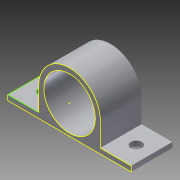
# Autodesk Inventor part: bearing mount
Saved by Autodesk Inventor 2013 (Build 170138000, 138)
## iProperties
Created: 2013-02-03
Part Number: bearing mount
Material: Aluminum 6061
Document SubType Name: Modeling
Designer: Arpan
Density: 2.71 g/cm^3
Mass: 38.247 g
Surface Area: 89.6456 cm^2
Volume: 14.1133 cm^3
Author: Arpan
Autodesk Inventor part; units mm, degrees
ref_plane "YZ Plane" through (0, 0, 0) normal (1, 0, 0) x (0, 1, 0)
ref_plane "XZ Plane" through (0, 0, 0) normal (0, 1, 0) x (-1, 0, 0)
ref_plane "XY Plane" through (0, 0, 0) normal (0, 0, 1) x (1, 0, 0)
sketch "Sketch1" plane through (0, 0, 0) normal (0, 0, 1) x (1, 0, 0)
  line L0 (0, 0) -> (-38.1, 0)
  line L1 (0, 0) -> (38.1, 0)
  line L2 (38.1, 0) -> (38.1, 3.175)
  line L3 (38.1, 3.175) -> (-38.1, 3.175)
  line L4 (-38.1, 3.175) -> (-38.1, 0)
  line L5 (0, 0) -> (0, 17.4625)
  circle A0 centre (0, 17.4625) radius 15.875
  arc A1 (7.6134, 0) -> (-7.6134, 0) centre (0, 17.4625) ccw
  line L6 (-19.05, 17.4625) -> (-19.05, 3.175)
  line L7 (19.05, 17.4625) -> (19.05, 3.175)
  dimension "d0" = 38.1
  dimension "d1" = 38.1
  dimension "d2" = 3.175
  dimension "d3" = 17.4625
  dimension "d4" = 31.75
  dimension "d5" = 3.175
  constraints: 16 end point, 4 perpendicular, 4 point on circle, 4 point on line, 2 centre point, 2 parallel, 2 tangent, 1 coincident, 1 collinear, 1 horizontal
  measures "d0" distance of L0.start L0.end
  measures "d1" distance of L0.start L1.end
  measures "d2" distance of L1.end L2.end
  measures "d3" distance of L0.start L5.end
  measures "d4" diameter of A0
  measures "d5" radial gap between concentric circles of A0 A1
extrude "Extrusion1" add sketch "Sketch1" along normal blind 25.4 contours L5 A0 L3 A1 L1 | L0 A1 L3 A0 L5 | L0 L4 L3 A1 | A1 L3 L2 L1 | A1 L3 A0 | L3 L6 A1 | A1 L7 L3
sketch "Sketch2" plane through (19.05, 3.175, 0) normal (0, 1, 0) x (1, 0, 0)
  line L0 (19.05, 0) -> (19.05, -25.4) projected
  line L1 (19.05, -12.7) -> (9.525, -12.7)
  circle A0 centre (9.525, -12.7) radius 3.3782
  line L2 (-57.15, 0) -> (-57.15, -25.4) projected
  line L3 (-38.1, 0) -> (-38.1, -25.4) projected
  line L4 (-57.15, -12.7) -> (-47.625, -12.7)
  circle A1 centre (-47.625, -12.7) radius 3.3782
  point P0 (-19.05, 0)
  dimension "d8" = 6.7564
  dimension "d13" = 9.525
  dimension "d14" = 6.7564
  dimension "d15" = 9.525
  constraints: 4 end point, 2 centre point, 2 coincident, 2 midpoint, 2 perpendicular
  measures "d8" diameter of A0
  measures "d13" distance of L4.start L4.end
  measures "d14" diameter of A1
  measures "d15" distance of L1.start L1.end
extrude "Extrusion2" cut sketch "Sketch2" against normal blind 25.4
sketch "Sketch3" plane through (0, 0, 25.4) normal (0, 0, 1) x (1, 0, 0)
  circle A0 centre (0, 17.4625) radius 15.875 projected
  line L0 (-38.1, 0) -> (38.1, 0) projected
  line L1 (38.1, 0) -> (38.1, 3.175) projected
  line L2 (38.1, 3.175) -> (19.05, 3.175) projected
  line L3 (19.05, 3.175) -> (19.05, 17.4625) projected
  arc A1 (19.05, 17.4625) -> (-19.05, 17.4625) centre (0, 17.4625) ccw projected
  line L4 (-19.05, 17.4625) -> (-19.05, 3.175) projected
  line L5 (-19.05, 3.175) -> (-38.1, 3.175) projected
  line L6 (-38.1, 3.175) -> (-38.1, 0) projected
  point P0 (0, 0)
sketch "Sketch4" plane through (-38.1, 3.175, 0) normal (0, 1, 0) x (1, 0, 0)
  circle A0 centre (9.525, -12.7) radius 3.3782 projected
  line L0 (19.05, 0) -> (0, 0) projected
  line L1 (0, 0) -> (0, -25.4) projected
  line L2 (19.05, -25.4) -> (0, -25.4) projected
  line L3 (19.05, 0) -> (19.05, -25.4) projected
  point P0 (38.1, 0)
sketch "Sketch5" plane through (-38.1, 3.175, 0) normal (0, 1, 0) x (1, 0, 0)
  circle A0 centre (9.525, -12.7) radius 3.3782
  line L0 (19.05, 0) -> (0, 0)
  line L1 (0, 0) -> (0, -25.4)
  line L2 (19.05, -25.4) -> (0, -25.4)
  line L3 (19.05, 0) -> (19.05, -25.4)
  point P0 (38.1, 0)
  constraints: 8 end point, 1 centre point
body "Solid1"
